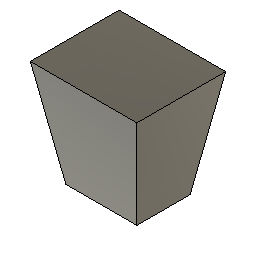
Cat_feeder_Case (Autodesk Fusion 360 design; units mm, degrees)
part number: 2026-05-04-17-01-12-873
part number: 2026-05-04-17-14-49-313
part number: 2026-05-04-17-15-05-830
part number: 2026-05-04-17-15-46-741
part number: 2026-05-04-17-16-01-391
Autodesk Fusion 360 part; units mm, degrees
sketch "Sketch1" plane through (0, 0, 0) normal (0, 0, 1) x (1, 0, 0)
sketch "Sketch1 (2)" plane through (0, 0, 0) normal (0, 0, 1) x (1, 0, 0) in component "Hopper"
  line L0 (60, -50) -> (-60, -50)
  line L1 (-60, -50) -> (-60, 50)
  line L2 (-60, 50) -> (60, 50)
  line L3 (60, 50) -> (60, -50)
  line L4 (60, -50) -> (-60, 50) construction
  line L5 (-60, -50) -> (60, 50) construction
  dimension "d1" = 120
  dimension "d2" = 100
  constraint horizontal L0
  constraint perpendicular L0 L1
  constraint parallel L0 L2
  constraint parallel L1 L3
  constraint coincident L4 origin
  constraint coincident L5 origin
  measures "d1" distance of L1.end L2.end
  measures "d2" distance of L0.end L1.end
ref_plane "WorkPlane1" through (0, 0, -120) normal (0, 0, 1) x (1, 0, 0) in component "Hopper"
sketch "Sketch2" plane through (0, 0, -120) normal (0, 0, 1) x (1, 0, 0) in component "Hopper"
  line L0 (40, 30) -> (-40, 30)
  line L1 (-40, 30) -> (-40, -30)
  line L2 (-40, -30) -> (40, -30)
  line L3 (40, -30) -> (40, 30)
  line L4 (40, 30) -> (-40, -30) construction
  line L5 (-40, 30) -> (40, -30) construction
  dimension "d4" = 80
  dimension "d5" = 60
  constraint horizontal L0
  constraint perpendicular L0 L1
  constraint parallel L0 L2
  constraint parallel L1 L3
  constraint coincident L4 origin
  constraint coincident L5 origin
  measures "d4" distance of L1.end L2.end
  measures "d5" distance of L0.end L1.end
loft "Loft1" add profiles "Sketch1 (2)", "Sketch2" section 1 section 2 in component "Hopper"
component "Hopper" placed x (1, 0, 0) y (0, 1, 0) z (0, 0, 1) at (0, 0, 0)
component "Main body" placed x (1, 0, 0) y (0, 1, 0) z (0, 0, 1) at (0, 0, 0)
component "Door" placed x (1, 0, 0) y (0, 1, 0) z (0, 0, 1) at (0, 0, 0)
component "Bowl" placed x (1, 0, 0) y (0, 1, 0) z (0, 0, 1) at (0, 0, 0)
